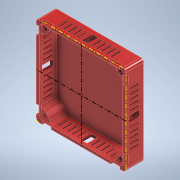
# Autodesk Inventor part: Led behuizing
Saved by Autodesk Inventor 2021 (Build 250183000, 183)
## iProperties
Created: 2023-10-02
Part Number: Led behuizing
Material: Generic
Document SubType Name: Modeling
Designer: Elias
Density: 1 g/cm^3
Appearance: Orange-Red
Author: Elias
Autodesk Inventor part; units mm, degrees
ref_plane "YZ Plane" through (0, 0, 0) normal (1, 0, 0) x (0, 1, 0)
ref_plane "XZ Plane" through (0, 0, 0) normal (0, 1, 0) x (-1, 0, 0)
ref_plane "XY Plane" through (0, 0, 0) normal (0, 0, 1) x (1, 0, 0)
sketch "Sketch1" plane through (0, 0, 0) normal (0, 0, 1) x (1, 0, 0)
  line L0 (0, 0) -> (150, 0)
  line L1 (150, 0) -> (150, 150)
  line L2 (150, 150) -> (0, 150)
  line L3 (0, 150) -> (0, 0)
  dimension "d0" = 150
  dimension "d1" = 150
  constraints: 8 end point, 2 parallel, 1 horizontal, 1 perpendicular
  measures "d0" distance of L2.end L1.end
  measures "d1" distance of L0.end L1.end
extrude "Extrusion1" add sketch "Sketch1" along normal blind 30
sketch "Sketch2" plane through (0, 0, 30) normal (0, 0, 1) x (1, 0, 0)
  line L0 (145, 130) -> (145, 20)
  line L1 (130, 5) -> (20, 5)
  line L2 (5, 20) -> (5, 130)
  line L3 (150, 150) -> (0, 150) projected
  line L4 (150, 0) -> (150, 150) projected
  arc A0 (145, 20) -> (130, 5) centre (145, 5) ccw
  line L5 (0, 150) -> (0, 0) projected
  line L6 (0, 75) -> (150, 75)
  line L7 (75, 150) -> (75, 0)
  line L8 (0, 0) -> (150, 0) projected
  arc A1 (20, 5) -> (5, 20) centre (5, 5) ccw
  arc A2 (5, 130) -> (20, 145) centre (5, 145) ccw
  arc A3 (130, 145) -> (145, 130) centre (145, 145) ccw
  line L9 (-10, 145) -> (0, 145)
  line L10 (20, 145) -> (130, 145)
  dimension "d5" = 5
  dimension "d6" = 140
  dimension "d10" = 15
  dimension "d11" = 5
  constraints: 14 end point, 9 symmetric about line, 8 point on circle, 4 centre point, 4 midpoint, 3 parallel, 2 horizontal, 2 perpendicular, 1 point on line, 3 other
  measures "d5" distance between parallel lines of L4 L0
  measures "d6" distance of L9.start L10.end
  measures "d10" radius of A0
  measures "d11" distance between parallel lines of L3 L10
extrude "Extrusion2" cut sketch "Sketch2" against normal blind 29.5 contours L0 L6 L7 L10 A3 | L0 A0 L1 L7 L6 | L7 L1 A1 L2 L6 | L6 L2 A2 L10 L7
fillet "Fillet1" radius 5 4 edges at (150, 150, 15) (150, 0, 15) (0, 150, 15) (0, 0, 15)
sketch "Sketch3" plane through (0, 0, 30) normal (0, 0, 1) x (1, 0, 0)
  line L0 (10, 145) -> (140, 145)
  line L1 (145, 140) -> (145, 10)
  line L2 (140, 5) -> (10, 5)
  line L3 (5, 10) -> (5, 140)
  line L4 (0, 145) -> (0, 5) projected
  line L5 (5, 0) -> (145, 0) projected
  arc A0 (10, 145) -> (5, 140) centre (10, 140) ccw
  arc A1 (145, 140) -> (140, 145) centre (140, 140) ccw
  arc A2 (140, 5) -> (145, 10) centre (140, 10) ccw
  arc A3 (5, 10) -> (10, 5) centre (10, 10) ccw
  point P0 (0, 0)
  point P1 (5, 145)
  point P2 (145, 5)
  point P3 (145, 145)
  dimension "d12" = 140
  dimension "d13" = 140
  dimension "d14" = 5
  dimension "d15" = 5
  dimension "d16" = 5
  constraints: 8 end point, 8 point on circle, 8 tangent, 6 point on line, 4 centre point, 3 equal radius, 2 parallel, 1 horizontal, 1 perpendicular
  measures "d12" distance of point (5, 145) point (145, 145)
  measures "d13" distance of point (145, 145) point (145, 5)
  measures "d14" distance between parallel lines of L4 L3
  measures "d15" distance between parallel lines of L5 L2
  measures "d16" radius of A0
extrude "Extrusion3" cut sketch "Sketch3" against normal blind 3
sketch "Sketch4" plane through (0, 0, 27) normal (0, 0, 1) x (1, 0, 0)
  line L0 (145, 150) -> (5, 150) projected
  line L1 (0, 145) -> (0, 5) projected
  line L2 (150, 5) -> (150, 145) projected
  line L3 (5, 0) -> (145, 0) projected
  point P0 (0, 0)
  point P1 (11.5, 138.5)
  point P2 (138.5, 138.5)
  point P3 (138.5, 11.5)
  point P4 (11.5, 11.5)
  dimension "d26" = 11.5
  dimension "d27" = 11.5
  dimension "d28" = 11.5
  dimension "d29" = 11.5
  dimension "d30" = 11.5
  dimension "d31" = 11.5
  dimension "d32" = 11.5
  dimension "d33" = 11.5
  measures "d26" distance from line of L0 point (11.5, 138.5)
  measures "d27" distance from line of L1 point (11.5, 138.5)
  measures "d28" distance from line of L0 point (138.5, 138.5)
  measures "d29" distance from line of L2 point (138.5, 138.5)
  measures "d30" distance from line of L2 point (138.5, 11.5)
  measures "d31" distance from line of L3 point (138.5, 11.5)
  measures "d32" distance from line of L3 point (11.5, 11.5)
  measures "d33" distance from line of L1 point (11.5, 11.5)
hole "Hole1" at (11.5, 138.5, 27) at (138.5, 138.5, 27) at (138.5, 11.5, 27) at (11.5, 11.5, 27) direction (0, 0, -1) diameter 8.2 depth 15
fillet "Fillet2" radius 5 8 edges at (20, 5, 13.75) (5, 20, 13.75) (5, 130, 13.75) (20, 145, 13.75) (130, 145, 13.75) (145, 130, 13.75) (130, 5, 13.75) (145, 20, 13.75)
sketch "Sketch5" plane through (5, 150, 0) normal (0, 1, 0) x (1, 0, 0)
  line L0 (25, -7) -> (28, -7)
  line L1 (28, -7) -> (28, -25)
  line L2 (28, -25) -> (25, -25)
  line L3 (25, -25) -> (25, -7)
  line L4 (140, -30) -> (0, -30) projected
  line L5 (-5, 0) -> (-5, -30) projected
  dimension "d35" = 3
  dimension "d36" = 18
  dimension "d37" = 5
  dimension "d38" = 30
  constraints: 8 end point, 2 parallel, 1 horizontal, 1 perpendicular
  measures "d35" distance of L1.end L2.end
  measures "d36" distance of L0.end L1.end
  measures "d37" distance between parallel lines of L4 L2
  measures "d38" distance between parallel lines of L3 L5
extrude "Extrusion4" cut sketch "Sketch5" against normal blind 10
pattern_linear "Rectangular Pattern1" count 12 spacing 8 along (1, 0, 0) of "Extrusion4"
sketch "Sketch7" plane through (150, 5, 0) normal (1, 0, 0) x (0, 0, -1)
  line L0 (-7, 115) -> (-25, 115)
  line L1 (-25, 115) -> (-25, 112)
  line L2 (-25, 112) -> (-7, 112)
  line L3 (-7, 112) -> (-7, 115)
  line L4 (-30, 0) -> (-30, 140) projected
  line L5 (0, 145) -> (-30, 145) projected
  point P0 (0, -5)
  dimension "d46" = 18
  dimension "d47" = 3
  dimension "d48" = 5
  dimension "d49" = 30
  constraints: 8 end point, 2 parallel, 1 horizontal, 1 perpendicular
  measures "d46" distance of L2.end L1.end
  measures "d47" distance of L2.end L0.start
  measures "d48" distance between parallel lines of L4 L1
  measures "d49" distance between parallel lines of L5 L0
extrude "Extrusion5" cut sketch "Sketch7" against normal blind 10
pattern_linear "Rectangular Pattern2" count 12 spacing 8 along (0, -1, 0) of "Extrusion5"
sketch "Sketch8" plane through (5, 0, 0) normal (0, -1, 0) x (1, 0, 0)
  line L0 (115, 7) -> (112, 7)
  line L1 (112, 7) -> (112, 25)
  line L2 (112, 25) -> (115, 25)
  line L3 (115, 25) -> (115, 7)
  line L4 (0, 30) -> (140, 30) projected
  line L5 (145, 0) -> (145, 30) projected
  point P0 (-5, 0)
  dimension "d55" = 3
  dimension "d56" = 5
  dimension "d57" = 30
  dimension "d58" = 18
  constraints: 8 end point, 2 parallel, 1 horizontal, 1 perpendicular
  measures "d55" distance of L1.end L2.end
  measures "d56" distance between parallel lines of L4 L2
  measures "d57" distance between parallel lines of L5 L3
  measures "d58" distance of L0.end L1.end
extrude "Extrusion6" cut sketch "Sketch8" against normal blind 10
pattern_linear "Rectangular Pattern3" count 12 spacing 8 along (-1, 0, 0) of "Extrusion6"
sketch "Sketch9" plane through (0, 5, 0) normal (-1, 0, 0) x (0, 0, 1)
  line L0 (25, 28) -> (7, 28)
  line L1 (7, 28) -> (7, 25)
  line L2 (7, 25) -> (25, 25)
  line L3 (25, 25) -> (25, 28)
  line L4 (30, 140) -> (30, 0) projected
  line L5 (0, -5) -> (30, -5) projected
  dimension "d64" = 3
  dimension "d65" = 18
  dimension "d66" = 5
  dimension "d67" = 30
  constraints: 8 end point, 2 parallel, 1 horizontal, 1 perpendicular
  measures "d64" distance of L0.end L1.end
  measures "d65" distance of L1.end L2.end
  measures "d66" distance between parallel lines of L4 L3
  measures "d67" distance between parallel lines of L5 L2
extrude "Extrusion7" cut sketch "Sketch9" against normal blind 10
pattern_linear "Rectangular Pattern4" count 12 spacing 8 along (0, 1, 0) of "Extrusion7"
sketch "Sketch11" plane through (0, 0, 30) normal (0, 0, 1) x (1, 0, 0)
  line L0 (150, 5) -> (150, 145) projected
  line L1 (150, 75) -> (0, 75)
  line L2 (145, 150) -> (5, 150) projected
  line L3 (75, 150) -> (75, 0)
  point P0 (0, 0)
  constraints: 4 end point, 2 midpoint, 1 horizontal, 1 vertical
sketch "Sketch10" plane through (0, 0, 30) normal (0, 0, 1) x (1, 0, 0)
  line L0 (140, 4) -> (125, 4)
  line L1 (125, 4) -> (125, 1)
  line L2 (125, 1) -> (140, 1)
  line L3 (140, 1) -> (140, 4)
  line L4 (0, 145) -> (0, 5) projected
  line L5 (5, 0) -> (145, 0) projected
  line L6 (140, 149) -> (125, 149)
  line L7 (125, 149) -> (125, 146)
  line L8 (125, 146) -> (140, 146)
  line L9 (140, 146) -> (140, 149)
  line L10 (150, 5) -> (150, 145) projected
  line L11 (145, 150) -> (5, 150) projected
  line L12 (25, 4) -> (10, 4)
  line L13 (10, 4) -> (10, 1)
  line L14 (10, 1) -> (25, 1)
  line L15 (25, 1) -> (25, 4)
  line L16 (25, 149) -> (10, 149)
  line L17 (10, 149) -> (10, 146)
  line L18 (10, 146) -> (25, 146)
  line L19 (25, 146) -> (25, 149)
  line L20 (146, 140) -> (149, 140)
  line L21 (149, 140) -> (149, 125)
  line L22 (149, 125) -> (146, 125)
  line L23 (146, 125) -> (146, 140)
  line L24 (145, 140) -> (145, 10) projected
  line L25 (146, 25) -> (149, 25)
  line L26 (149, 25) -> (149, 10)
  line L27 (149, 10) -> (146, 10)
  line L28 (146, 10) -> (146, 25)
  line L29 (1, 140) -> (4, 140)
  line L30 (4, 140) -> (4, 125)
  line L31 (4, 125) -> (1, 125)
  line L32 (1, 125) -> (1, 140)
  line L33 (1, 25) -> (4, 25)
  line L34 (4, 25) -> (4, 10)
  line L35 (4, 10) -> (1, 10)
  line L36 (1, 10) -> (1, 25)
  point P0 (0, 0)
  dimension "d75" = 3
  dimension "d76" = 15
  dimension "d77" = 125
  dimension "d78" = 1
  dimension "d81" = 15
  dimension "d82" = 3
  dimension "d83" = 10
  dimension "d84" = 1
  dimension "d85" = 15
  dimension "d86" = 3
  dimension "d87" = 10
  dimension "d88" = 1
  dimension "d89" = 3
  dimension "d90" = 15
  dimension "d91" = 10
  dimension "d92" = 1
  dimension "d93" = 3
  dimension "d94" = 15
  dimension "d95" = 1
  dimension "d96" = 10
  dimension "d97" = 15
  dimension "d98" = 3
  dimension "d99" = 1
  dimension "d100" = 10
  dimension "d101" = 3
  dimension "d102" = 15
  dimension "d103" = 1
  dimension "d104" = 10
  dimension "d105" = 3
  dimension "d106" = 1
  dimension "d107" = 10
  dimension "d108" = 15
  constraints: 64 end point, 16 parallel, 8 horizontal, 8 perpendicular
  measures "d75" distance of L0.end L1.end
  measures "d76" distance of L1.end L2.end
  measures "d77" distance between parallel lines of L1 L4
  measures "d78" distance between parallel lines of L5 L2
  measures "d81" distance of L7.end L8.end
  measures "d82" distance of L8.end L6.start
  measures "d83" distance between parallel lines of L10 L9
  measures "d84" distance between parallel lines of L11 L6
  measures "d85" distance of L13.end L14.end
  measures "d86" distance of L12.end L13.end
  measures "d87" distance between parallel lines of L4 L13
  measures "d88" distance between parallel lines of L5 L14
  measures "d89" distance of L18.end L16.start
  measures "d90" distance of L17.end L18.end
  measures "d91" distance between parallel lines of L4 L17
  measures "d92" distance between parallel lines of L11 L16
  measures "d93" distance of L20.start L20.end
  measures "d94" distance of L22.end L20.start
  measures "d95" distance between parallel lines of L24 L23
  measures "d96" distance between parallel lines of L11 L20
  measures "d97" distance of L25.end L26.end
  measures "d98" distance of L26.end L27.end
  measures "d99" distance between parallel lines of L10 L26
  measures "d100" distance between parallel lines of L5 L27
  measures "d101" distance of L33.start L33.end
  measures "d102" distance of L35.end L33.start
  measures "d103" distance between parallel lines of L4 L36
  measures "d104" distance between parallel lines of L5 L35
  measures "d105" distance of L29.start L29.end
  measures "d106" distance between parallel lines of L4 L32
  measures "d107" distance between parallel lines of L11 L29
  measures "d108" distance of L31.end L29.start
extrude "Extrusion8" cut sketch "Sketch10" against normal blind 15
sketch "Sketch12" plane through (5, 150, 0) normal (0, 1, 0) x (1, 0, 0)
  line L0 (5, -30) -> (5, -27) projected
  line L1 (5, -30) -> (5, -26)
  line L2 (5, -26) -> (20, -26)
  line L3 (20, -26) -> (20, -30)
  line L4 (140, -30) -> (0, -30) projected
  line L5 (5, -30) -> (20, -30)
  line L6 (135, -30) -> (135, -27) projected
  line L7 (135, -30) -> (135, -26)
  line L8 (135, -26) -> (120, -26)
  line L9 (120, -30) -> (120, -15) projected
  line L10 (120, -26) -> (120, -30)
  line L11 (135, -30) -> (5, -30) projected
  line L12 (120, -30) -> (135, -30)
  point P0 (-5, 0)
  dimension "d109" = 4
  dimension "d110" = 15
  dimension "d113" = 4
  dimension "d114" = 15
  constraints: 16 end point, 4 perpendicular, 3 point on line, 1 collinear
  measures "d109" distance of L0.start L1.end
  measures "d110" distance of L1.end L2.end
  measures "d113" distance of L6.start L7.end
  measures "d114" distance of L7.end L8.end
extrude "Extrusion9" cut sketch "Sketch12" against normal blind 2
sketch "Sketch13" plane through (150, 5, 0) normal (1, 0, 0) x (0, 0, -1)
  line L0 (-30, 5) -> (-15, 5) projected
  line L1 (-30, 5) -> (-26, 5)
  line L2 (-26, 5) -> (-26, 20)
  line L3 (-30, 20) -> (-15, 20) projected
  line L4 (-26, 20) -> (-30, 20)
  line L5 (-30, 20) -> (-30, 5) projected
  line L6 (-30, 20) -> (-30, 5)
  line L7 (-30, 135) -> (-15, 135) projected
  line L8 (-30, 135) -> (-26, 135)
  line L9 (-26, 135) -> (-26, 120)
  line L10 (-30, 120) -> (-15, 120) projected
  line L11 (-26, 120) -> (-30, 120)
  line L12 (-30, 120) -> (-30, 135)
  point P0 (0, -5)
  dimension "d115" = 4
  dimension "d116" = 15
  dimension "d117" = 4
  dimension "d118" = 15
  constraints: 16 end point, 2 perpendicular, 2 point on line, 1 collinear
  measures "d115" distance of L0.start L1.end
  measures "d116" distance of L1.end L2.end
  measures "d117" distance of L7.start L8.end
  measures "d118" distance of L8.end L9.end
extrude "Extrusion10" cut sketch "Sketch13" against normal blind 2
sketch "Sketch14" plane through (0, 5, 0) normal (-1, 0, 0) x (0, 0, 1)
  line L0 (30, 120) -> (30, 135) projected
  line L1 (26, 135) -> (15, 135) projected
  line L2 (30, 135) -> (26, 135)
  line L3 (26, 135) -> (26, 120) projected
  line L4 (26, 135) -> (26, 120)
  line L5 (30, 120) -> (15, 120) projected
  line L6 (26, 120) -> (30, 120)
  line L7 (30, 140) -> (30, 135) projected
  line L8 (30, 120) -> (30, 135)
  line L9 (30, 5) -> (30, 20) projected
  line L10 (30, 5) -> (26, 5)
  line L11 (30, 5) -> (15, 5) projected
  line L12 (26, 5) -> (26, 20)
  line L13 (26, 20) -> (30, 20)
  line L14 (30, 20) -> (30, 5)
  point P0 (0, -5)
  dimension "d121" = 4
  dimension "d122" = 4
  dimension "d123" = 15
  constraints: 16 end point, 5 perpendicular, 2 collinear, 1 point on line
  measures "d121" distance of L0.end L1.start
  measures "d122" distance of L9.start L10.end
  measures "d123" distance of L10.end L12.end
extrude "Extrusion11" cut sketch "Sketch14" against normal blind 2
sketch "Sketch15" plane through (5, 0, 0) normal (0, -1, 0) x (1, 0, 0)
  line L0 (5, 30) -> (5, 27) projected
  line L1 (5, 30) -> (5, 26)
  line L2 (5, 26) -> (20, 26)
  line L3 (20, 30) -> (20, 15) projected
  line L4 (20, 26) -> (20, 30)
  line L5 (0, 30) -> (5, 30) projected
  line L6 (20, 30) -> (5, 30)
  line L7 (135, 26) -> (120, 26) projected
  line L8 (135, 30) -> (135, 26)
  line L9 (135, 26) -> (120, 26)
  line L10 (120, 26) -> (120, 30)
  line L11 (135, 30) -> (120, 30) projected
  line L12 (120, 30) -> (135, 30)
  point P0 (-5, 0)
  dimension "d126" = 4
  dimension "d127" = 15
  constraints: 16 end point, 3 collinear, 2 perpendicular, 2 point on line, 1 vertical
  measures "d126" distance of L0.start L1.end
  measures "d127" distance of L1.end L2.end
extrude "Extrusion12" cut sketch "Sketch15" against normal blind 2
fillet "Fillet3" radius 1 8 edges at (149, 132.5, 26) (149, 17.5, 26) (132.5, 1, 26) (17.5, 1, 26) (1, 17.5, 26) (1, 132.5, 26) (17.5, 149, 26) (132.5, 149, 26)
sketch "Sketch17" plane through (5, 0, 0) normal (0, -1, 0) x (1, 0, 0)
  line L0 (67, 25) -> (67, 7) projected
  line L1 (67, 25) -> (72, 25)
  line L2 (72, 7) -> (72, 25) projected
  line L3 (72, 25) -> (72, 7)
  line L4 (67, 7) -> (64, 7) projected
  line L5 (72, 7) -> (67, 7)
  line L6 (67, 7) -> (67, 25)
  point P0 (-5, 0)
  constraints: 8 end point, 2 perpendicular, 1 collinear
extrude "Extrusion13" cut sketch "Sketch17" against normal blind 10
sketch "Sketch18" plane through (150, 5, 0) normal (1, 0, 0) x (0, 0, -1)
  line L0 (-7, 67) -> (-25, 67) projected
  line L1 (-25, 72) -> (-7, 72) projected
  line L2 (-25, 67) -> (-25, 72)
  line L3 (-25, 72) -> (-7, 72)
  line L4 (-25, 67) -> (-7, 67)
  line L5 (-7, 72) -> (-7, 67)
  point P0 (0, -5)
  constraints: 8 end point, 2 perpendicular, 1 collinear
extrude "Extrusion14" cut sketch "Sketch18" against normal blind 10
sketch "Sketch19" plane through (5, 150, 0) normal (0, 1, 0) x (1, 0, 0)
  line L0 (73, -7) -> (73, -25) projected
  line L1 (68, -25) -> (68, -7) projected
  line L2 (73, -25) -> (68, -25)
  line L3 (68, -25) -> (68, -7)
  line L4 (68, -7) -> (73, -7)
  line L5 (64, -7) -> (75, -7) projected
  point P0 (-5, 0)
  constraints: 6 end point, 1 collinear, 1 perpendicular, 1 point on line
extrude "Extrusion15" cut sketch "Sketch19" against normal blind 10
sketch "Sketch20" plane through (0, 5, 0) normal (-1, 0, 0) x (0, 0, 1)
  line L0 (25, 76) -> (25, 73) projected
  line L1 (25, 68) -> (7, 68) projected
  line L2 (25, 73) -> (25, 68)
  line L3 (25, 73) -> (7, 73) projected
  line L4 (25, 73) -> (7, 73)
  line L5 (7, 73) -> (7, 68)
  point P0 (0, -5)
  constraints: 6 end point, 1 collinear, 1 perpendicular, 1 vertical
extrude "Extrusion16" cut sketch "Sketch20" against normal blind 10
body "Solid1"
